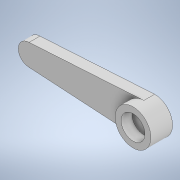
# Autodesk Inventor part: servo-swap
Saved by Autodesk Inventor 2021 (Build 250183000, 183)
## iProperties
Created: 2024-04-27
Part Number: servo-swap
Material: Generic
Document SubType Name: Modeling
Designer: Toby
Density: 1 g/cm^3
Appearance: Default
Author: Toby
Autodesk Inventor part; units mm, degrees
ref_plane "YZ Plane" through (0, 0, 0) normal (1, 0, 0) x (0, 1, 0)
ref_plane "XZ Plane" through (0, 0, 0) normal (0, 1, 0) x (-1, 0, 0)
ref_plane "XY Plane" through (0, 0, 0) normal (0, 0, 1) x (1, 0, 0)
sketch "Sketch1" plane through (0, 0, 0) normal (0, 0, 1) x (1, 0, 0)
  circle A0 centre (0, 0) radius 3.3
  circle A1 centre (-21.2, 0) radius 2
  line L0 (-21.2, 2) -> (0, 3.3)
  line L1 (0, -3.3) -> (-21.2, -2)
  dimension "d0" = 6.6
  dimension "d1" = 4
  dimension "d2" = 21.2
  constraints: 4 end point, 4 point on circle, 2 centre point, 1 coincident
  measures "d0" diameter of A0
  measures "d1" diameter of A1
  measures "d2" distance of point (0, 0) A1.centre
extrude "Extrusion1" add sketch "Sketch1" along normal blind 2 contours A0 L1 L0 | A0 L1 A1 L0 | A1
sketch "Sketch2" plane through (0, 0, 2) normal (0, 0, 1) x (1, 0, 0)
  arc A0 (0, -3.3) -> (0, 3.3) centre (0, 0) ccw projected
  circle A1 centre (0, 0) radius 3.3
  circle A2 centre (0, 0) radius 2.2
  dimension "d5" = 4.4
  constraints: 2 coincident, 1 centre point, 3 other
  measures "d5" diameter of A2
extrude "Extrusion2" add sketch "Sketch2" along normal blind 2
body "Solid1"
